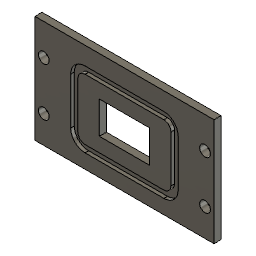
metal plate swap (Autodesk Fusion 360 design; units mm, degrees)
part number: 2026-04-01-23-45-42-025
Autodesk Fusion 360 part; units mm, degrees
note: some values were not read from the file. Set by a fixed rule: which sketch regions a step uses.
sketch "Sketch1" plane through (0, 0, 0) normal (0, 0, 1) x (1, 0, 0)
  line L0 (0, 0) -> (50, 0)
  line L1 (50, 0) -> (50, 27)
  line L2 (50, 27) -> (0, 27)
  line L3 (0, 27) -> (0, 0)
  dimension "d1" = 27
  dimension "d2" = 50
  constraint horizontal L0
  constraint vertical L1
  constraint horizontal L2
  constraint vertical L3
  constraint coincident L0.start L3.end
  measures "d1" distance of L0.start L2.end
  measures "d2" distance of L0.start L0.end
extrude "Extrude1" add sketch "Sketch1" against normal blind 5
extrude "Extrude2" cut 1 faces at (16.6667, 18, -5) along direction (0, 0, 1) blind 3
sketch "Sketch3" plane through (0, 0, 0) normal (0, 0, 1) x (1, 0, 0)
  line L0 (0, 27) -> (0, 0)
  line L1 (0, 0) -> (50, 0)
  line L2 (50, 0) -> (50, 27)
  line L3 (50, 27) -> (0, 27)
  line L4 (10, 24) -> (40, 24)
  line L5 (40, 24) -> (40, 3)
  line L6 (40, 3) -> (10, 3)
  line L7 (10, 3) -> (10, 24)
  line L8 (36, 5) -> (14, 5)
  line L9 (12, 7) -> (12, 20)
  line L10 (14, 22) -> (36, 22)
  line L11 (38, 20) -> (38, 7)
  arc A0 (38, 20) -> (36, 22) centre (36, 20) ccw
  arc A1 (36, 5) -> (38, 7) centre (36, 7) ccw
  arc A2 (12, 7) -> (14, 5) centre (14, 7) ccw
  arc A3 (14, 22) -> (12, 20) centre (14, 20) ccw
  dimension "d10" = 21
  dimension "d11" = 3
  dimension "d12" = 30
  dimension "d13" = 10
  dimension "d22" = 2
  constraint horizontal L4
  constraint vertical L5
  constraint horizontal L6
  constraint vertical L7
  constraint tangent L10 A0
  constraint tangent L11 A0
  constraint tangent L8 A1
  constraint tangent L11 A1
  constraint equal A0 A1
  constraint tangent L8 A2
  constraint tangent L9 A2
  constraint equal A0 A2
  constraint tangent L9 A3
  constraint tangent L10 A3
  constraint equal A0 A3
  measures "d10" distance of L4.start L6.end
  measures "d11" distance of L3 L4
  measures "d12" distance of L5.end L6.end
  measures "d13" distance of L0 L7
  measures "d22" radius of A0
extrude "Extrude3" add 1 faces at (16.6667, 18, -2) along direction (0, 0, -1) blind 1
extrude "Extrude4" cut sketch "Sketch3" against normal blind 2 contours L8 L9 L10 L11 A0 A1 A2 A3
sketch "Sketch5" plane through (0, 0, 0) normal (0, 0, 1) x (1, 0, 0)
  line L0 (14, 22) -> (36, 22)
  arc A0 (38, 20) -> (36, 22) centre (36, 20) ccw
  line L1 (38, 20) -> (38, 7)
  arc A1 (36, 5) -> (38, 7) centre (36, 7) ccw
  line L2 (36, 5) -> (14, 5)
  arc A2 (12, 7) -> (14, 5) centre (14, 7) ccw
  line L3 (12, 7) -> (12, 20)
  arc A3 (14, 22) -> (12, 20) centre (14, 20) ccw
  line L4 (0, 27) -> (0, 0)
  line L5 (0, 0) -> (50, 0)
  line L6 (50, 0) -> (50, 27)
  line L7 (50, 27) -> (0, 27)
  line L8 (14, 24) -> (36, 24)
  arc A4 (40, 20) -> (36, 24) centre (36, 20) ccw
  line L9 (40, 20) -> (40, 7)
  arc A5 (36, 3) -> (40, 7) centre (36, 7) ccw
  line L10 (36, 3) -> (14, 3)
  arc A6 (10, 7) -> (14, 3) centre (14, 7) ccw
  line L11 (10, 7) -> (10, 20)
  arc A7 (14, 24) -> (10, 20) centre (14, 20) ccw
  dimension "d23" = 2
  measures "d23" distance of A0
extrude "Extrude5" cut sketch "Sketch5" against normal blind 1 contours L8 A4 L9 A5 L10 A6 L11 A7
sketch "Sketch6" plane through (0, 0, -2) normal (0, 0, 1) x (1, 0, 0)
  arc A0 (38, 20) -> (36, 22) centre (36, 20) ccw
  line L0 (36, 22) -> (14, 22)
  arc A1 (14, 22) -> (12, 20) centre (14, 20) ccw
  line L1 (12, 20) -> (12, 7)
  arc A2 (12, 7) -> (14, 5) centre (14, 7) ccw
  line L2 (14, 5) -> (36, 5)
  arc A3 (36, 5) -> (38, 7) centre (36, 7) ccw
  line L3 (38, 7) -> (38, 20)
  line L4 (18, 18) -> (32, 18)
  line L5 (32, 18) -> (32, 9)
  line L6 (32, 9) -> (18, 9)
  line L7 (18, 9) -> (18, 18)
  dimension "d28" = 4
  dimension "d29" = 4
  dimension "d30" = 9
  dimension "d31" = 6
  dimension "d32" = 6
  constraint horizontal L4
  constraint vertical L5
  constraint horizontal L6
  constraint vertical L7
  measures "d28" distance of L2 L6
  measures "d29" distance of L0 L4
  measures "d30" distance of L4.start L6.end
  measures "d31" distance of L3 L5
  measures "d32" distance of L1 L7
extrude "Extrude6" cut sketch "Sketch6" against normal blind 10 contours L4 L5 L6 L7
sketch "Sketch7" plane through (0, 0, 0) normal (0, 0, 1) x (1, 0, 0)
  line L0 (14, 24) -> (36, 24)
  arc A0 (40, 20) -> (36, 24) centre (36, 20) ccw
  line L1 (40, 20) -> (40, 7)
  arc A1 (36, 3) -> (40, 7) centre (36, 7) ccw
  line L2 (36, 3) -> (14, 3)
  arc A2 (10, 7) -> (14, 3) centre (14, 7) ccw
  line L3 (10, 7) -> (10, 20)
  arc A3 (14, 24) -> (10, 20) centre (14, 20) ccw
  line L4 (0, 27) -> (0, 0)
  line L5 (0, 0) -> (50, 0)
  line L6 (50, 0) -> (50, 27)
  line L7 (50, 27) -> (0, 27)
  line L8 (0, 27) -> (5, 27)
  line L9 (5, 27) -> (5, 0)
  line L10 (5, 13.5) -> (0, 13.5)
  line L11 (2.5, 13.5) -> (2.5, 27)
  line L12 (2.5, 13.5) -> (2.5, 20.25)
  circle A4 centre (2.5, 20.25) radius 1.5
  line L13 (2.5, 13.5) -> (2.5, 6.75)
  circle A5 centre (2.5, 6.75) radius 1.5
  line L14 (50, 27) -> (45, 27)
  line L15 (45, 27) -> (45, 0)
  line L16 (45, 0) -> (50, 0)
  line L17 (50, 0) -> (50, 27)
  line L18 (45, 13.5) -> (50, 13.5)
  line L19 (47.5, 13.5) -> (47.5, 20.25)
  circle A6 centre (47.5, 20.25) radius 1.5
  line L20 (47.5, 13.5) -> (47.5, 6.75)
  circle A7 centre (47.5, 6.75) radius 1.5
  dimension "d35" = 3
  dimension "d36" = 6.75
  dimension "d37" = 3
  dimension "d40" = 6.75
  dimension "d41" = 3
  dimension "d42" = 6.75
  dimension "d43" = 3
  constraint coincident L4.start L7.end
  constraint coincident L7 L8.end
  constraint coincident L5 L9.end
  constraint perpendicular L5 L9
  constraint midpoint L9 L10.start
  constraint midpoint L4 L10.end
  constraint midpoint L10 L11.start
  constraint midpoint L8 L11.end
  constraint midpoint L11 L12.end
  constraint coincident L12.end A4.centre
  constraint perpendicular L10 L13
  constraint coincident L13.end A5.centre
  constraint horizontal L14
  constraint vertical L15
  constraint horizontal L16
  constraint vertical L17
  constraint coincident L5 L15.end
  constraint coincident L6.end L7.start
  constraint midpoint L15 L18.start
  constraint midpoint L17 L18.end
  constraint midpoint L18 L19.start
  constraint perpendicular L18 L19
  constraint coincident L19.end A6.centre
  constraint perpendicular L18 L20
  constraint coincident L20.end A7.centre
  measures "d35" diameter of A4
  measures "d36" distance of L11.start L13.end
  measures "d37" diameter of A5
  measures "d40" distance of L19.start L19.end
  measures "d41" diameter of A6
  measures "d42" distance of L19.start L20.end
  measures "d43" diameter of A7
extrude "Extrude7" cut sketch "Sketch7" against normal blind 10 contours L11 L12 A4 | L11 L12 A4 | A5
extrude "Extrude8" cut sketch "Sketch7" against normal blind 11 contours L11 L12 A4 | L11 L12 A4 | A5 | A6 | A7
extrude "Extrude9" add 1 faces at (36, 15, -2) along direction (0, 0, 1) blind 2
extrude "Extrude10" cut 1 faces at (22.6667, 24, -3) along direction (0, 0, 1) blind 1
extrude "Extrude11" add 1 faces at (33.3333, 27, -0.6667) along direction (0, 1, 0) blind 2
extrude "Extrude12" add 1 faces at (16.6667, 0, -0.6667) along direction (0, -1, 0) blind 1
